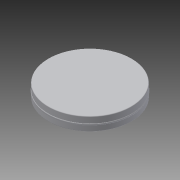
# Autodesk Inventor part: CaseBottom
Saved by Autodesk Inventor 2014 (Build 180170000, 170)
## iProperties
Created: 2014-11-03
Part Number: CaseBottom
Material: Polycarbonate, Smoke
Document SubType Name: Modeling
Designer: DV
Mass: 0.0593729 g
Surface Area: 7.41319 cm^2
Volume: 0.0494774 cm^3
Density: 1.2 g/cm^3
Appearance: Polycarbonate - Smoked
Author: DV
Autodesk Inventor part; units mm, degrees
ref_plane "YZ Plane" through (0, 0, 0) normal (1, 0, 0) x (0, 1, 0)
ref_plane "XZ Plane" through (0, 0, 0) normal (0, 1, 0) x (-1, 0, 0)
ref_plane "XY Plane" through (0, 0, 0) normal (0, 0, 1) x (1, 0, 0)
sketch "Sketch1" plane through (0, 0, 0) normal (0, 0, 1) x (1, 0, 0)
  line L0 (-8.4318, -121.1393) -> (-8.4318, -118.1834)
  line L1 (8.3829, -117.9353) -> (-8.3829, -117.9353)
  arc A0 (-8.3829, -117.9353) -> (-8.4318, -118.1834) centre (-8.3829, -118.0642) ccw
  line L2 (4.3376, -116.7353) -> (-7.8003, -116.7353) projected
  line L3 (0, -114.8242) -> (0, -125.5705)
  line L4 (-8.4421, -116.6072) -> (0, -116.6072)
  line L5 (0, -116.6072) -> (0, -119.3557)
  line L6 (-8.4318, -119.3546) -> (-8.4421, -119.3546)
  line L7 (-8.4318, -116.8623) -> (-8.4318, -119.3546)
  arc A1 (-8.5691, -117.8886) -> (-8.5691, -118.2397) centre (-8.3829, -118.0642) ccw
  line L8 (-8.5691, -119.2276) -> (-8.5691, -118.2397)
  line L9 (-8.5691, -117.8886) -> (-8.5691, -116.7342)
  line L10 (0, -116.7353) -> (-8.3048, -116.7353)
  arc A2 (-8.5691, -119.2276) -> (-8.4421, -119.3546) centre (-8.4421, -119.2276) ccw
  arc A3 (-8.3048, -116.7353) -> (-8.4318, -116.8623) centre (-8.3048, -116.8623) ccw
  arc A4 (-8.4421, -116.6072) -> (-8.5691, -116.7342) centre (-8.4421, -116.7342) ccw
  point P0 (0, 0)
  point P1 (0, -117.9353)
  dimension "d1" = 0.127
  dimension "d3" = 0.127
  constraints: 20 end point, 10 point on circle, 6 tangent, 5 centre point, 5 point on line, 3 horizontal, 3 parallel, 3 perpendicular, 2 equal radius, 1 coincident, 1 collinear, 1 midpoint, 1 vertical, 8 other
  measures "d1" radial gap between concentric circles of A1 A0
  measures "d3" radius of A2
revolve "Revolution1" add sketch "Sketch1" angle 360 about axis through (0, -114.8242, 0) along (0, -1, 0) contours L6 A2 L8 A1 L9 A4 L4 L3 L2 L10 A3 L7 A0 L0 | A0 L7
body "Solid1"
